potato_wall_hook (Autodesk Fusion 360 design; units mm, degrees)
Autodesk Fusion 360 part; units mm, degrees
sketch "Sketch1" plane through (0, 0, 0) normal (1, 0, 0) x (0, 1, 0)
  line L0 (0, 0) -> (10, 0)
  line L1 (10, 0) -> (10, 20)
  line L2 (10, 20) -> (0, 20)
  line L3 (0, 20) -> (0, 0)
  circle A0 centre (5, 14) radius 1.25
  line L4 (5, 20) -> (5, 0) construction
  dimension "d1" = 10
  dimension "d2" = 20
  dimension "d3" = 6
  dimension "d4" = 2.5
  constraint horizontal L0
  constraint vertical L1
  constraint horizontal L2
  constraint vertical L3
  constraint coincident L0.start L3.end
  constraint midpoint L2 L4.start
  constraint midpoint L0 L4.end
  constraint coincident A0.centre L4
  measures "d1" distance of L0.start L0.end
  measures "d2" distance of L0.end L1.end
  measures "d3" distance of L2 A0.centre
  measures "d4" diameter of A0
extrude "Extrude1" add sketch "Sketch1" along normal blind 4
ref_plane "WorkPlane1" through (0, 5, 0) normal (0, 1, 0) x (0, 0, 1)
sketch "Sketch2" plane through (0, 5, 0) normal (0, 1, 0) x (1, 0, 0)
  spline S0 degree 5 poles (4, 0) (4.5771, -0.1055) (5.7551, -0.2992) (7.5934, -0.5374) (10.1902, -0.7501) (13.6911, -0.8547) (17.4735, -0.8864) (21.5365, -0.9956) (25.924, -1.5675) (30.3819, -2.7889) (34.4435, -4.6461) (36.9623, -6.5714) (38.2422, -8.2146) (38.7971, -9.3913) (39, -10) knots 0 0 0 0 0 0 0.1 0.2 0.3 0.4 0.5 0.6 0.7 0.8 0.9 1 1 1 1 1 1
  line L0 (15.7367, -0.7193) -> (25.4307, -1.3448)
  line L1 (0, 0) -> (4, 0)
  line L2 (38, -7) -> (40, -13)
  spline S1 degree 5 poles (39, -10) (38.7242, -9.8626) (38.1556, -9.5847) (37.2514, -9.1586) (35.9422, -8.5717) (34.1308, -7.8106) (32.1444, -7.0347) (29.9895, -6.2707) (27.6837, -5.5654) (25.2519, -4.9777) (22.7222, -4.5714) (20.1223, -4.4064) (17.4768, -4.5309) (14.8034, -4.9704) (12.1137, -5.7332) (9.4148, -6.8176) (7.2511, -7.9369) (5.6263, -8.915) (4.5423, -9.6281) (4, -10) knots 0 0 0 0 0 0 0.066667 0.133333 0.2 0.266667 0.333333 0.4 0.466667 0.533333 0.6 0.666667 0.733333 0.8 0.866667 0.933333 1 1 1 1 1 1
  line L3 (4, 0) -> (4, -10)
  line L4 (39, -10) -> (30.4055, -5.1224)
  point P0 (20.5837, -1.0321)
  point P1 (32, -7)
  point P2 (19.692, -4.4795)
  dimension "d8" = 35
  dimension "d9" = 10
  dimension "d10" = 4
  dimension "d11" = 10
  constraint midpoint P0 L0
  constraint coincident L1.start origin
  constraint horizontal L1
  constraint coincident S0.start L1.end
  constraint midpoint S0.end L2
  constraint perpendicular L1 L3
  constraint coincident S1.end L3.end
  measures "d8" distance of S0.start S0.end
  measures "d9" distance of S0.start S0.end
  measures "d10" distance of L1.start S0.start
  measures "d11" distance of S0.start S1.end
extrude "Extrude2" add sketch "Sketch2" along normal mid plane 10
sketch "Sketch3" plane through (0, 0, 0) normal (0, 0, -1) x (1, 0, 0)
  line L0 (0, 0) -> (0, -10)
  line L1 (0, -10) -> (4, -10)
  line L2 (4, -10) -> (4, 0)
  line L3 (4, 0) -> (0, 0)
  line L4 (4, -10) -> (39.3, -7.5414)
  line L5 (39.3, -7.5414) -> (39.3, -2.5414)
  line L6 (39.3, -2.5414) -> (4, 0)
  line L7 (4, -10) -> (44.4178, -17.1605)
  line L8 (44.4178, -17.1605) -> (44.4178, 8.7922)
  line L9 (44.4178, 8.7922) -> (4, 0)
  dimension "d16" = 5
  dimension "d17" = 35.3
  constraint coincident L1.end L2.start
  constraint perpendicular L1 L5
  constraint coincident L2.end L3.start
  constraint perpendicular L1 L8
  measures "d16" distance of L4.end L5.end
  measures "d17" distance of L2 L5
extrude "Extrude3" cut sketch "Sketch3" against normal blind 15 contours L4 L5 L6 L7 L8 L9
ref_plane "WorkPlane2" through (39, 2.5199, 10) normal (-0.493575, 0, 0.869703) x (0, -1, 0)
sketch "Sketch4" plane through (5.2084, 0, -9.1775) normal (-0.493575, 0, 0.869703) x (0, -1, 0)
  line L0 (-7.5622, 38.8542) -> (-2.52, 38.8542)
  line L1 (-2.52, 38.8542) -> (-2.2042, 34.0638)
  line L2 (-2.2042, 34.0638) -> (-7.8675, 34.0638)
  line L3 (-7.8675, 34.0638) -> (-7.5622, 38.8542)
  constraint horizontal L0
  constraint parallel L0 L2
ref_plane "WorkPlane3" through (0, 0, 38) normal (0, 0, 1) x (1, 0, 0)
sketch "Sketch5" plane through (0, 0, 38) normal (0, 0, 1) x (1, 0, 0)
  circle A0 centre (37.674, 5.005) radius 1.25
  dimension "d25" = 2.5
  measures "d25" diameter of A0
loft "Loft1" add profiles "Sketch4", "Sketch5" section 1 section 2
